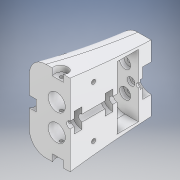
# Autodesk Inventor part: AA016
Saved by Autodesk Inventor 2017 SP1 (Build 210196100, 196)
## iProperties
Created: 2017-09-29
Part Number: AA016
Material: ABS Plastic
Document SubType Name: Modeling
Designer: Zach
Density: 1.06 g/cm^3
Appearance: CR White
Author: Zach
Autodesk Inventor part; units mm, degrees
sketch "Sketch1" plane through (0, 0, 0) normal (0, 0, 1) x (1, 0, 0)
  line L0 (0, 0) -> (70, 0)
  line L1 (70, 0) -> (70, 77.5)
  line L2 (70, 77.5) -> (0, 77.5)
  line L3 (0, 77.5) -> (0, 0)
  dimension "d0" = 70
  dimension "d1" = 77.5
  constraints: 8 end point, 2 parallel, 1 horizontal, 1 perpendicular
  measures "d0" distance of L2.end L1.end
  measures "d1" distance of L1.end L0.end
extrude "Extrusion1" add sketch "Sketch1" along normal blind 95
sketch "Sketch3" plane through (0, 0, 95) normal (0, 0, 1) x (1, 0, 0)
  line L0 (0, 0) -> (70, 0) projected
  line L1 (70, 77.5) -> (0, 77.5) projected
  line L2 (70, 0) -> (35, 0)
  line L3 (35, 0) -> (35, 77.5)
  line L4 (35, 77.5) -> (70, 77.5)
  line L5 (70, 77.5) -> (70, 0)
  constraints: 8 end point, 2 parallel, 1 horizontal, 1 midpoint, 1 perpendicular
extrude "Extrusion3" cut sketch "Sketch3" against normal through all
sketch "Sketch4" plane through (0, 77.5, 95) normal (0, 1, 0) x (1, 0, 0)
  line L0 (0, 95) -> (0, 0) projected
  line L1 (0, 0) -> (-12.5, 0)
  line L2 (35, 95) -> (0, 95) projected
  arc A0 (-12.5, 0) -> (0, 95) centre (-1145.4326, 197.3924) ccw
  line L3 (-12.5, -10) -> (35, -10) construction
  dimension "d9" = 1150
  dimension "d54" = 47.5
  dimension "d55" = 10
  constraints: 4 end point, 2 horizontal, 2 point on circle, 2 vertical alignment, 1 centre point
  measures "d9" radius of A0
  measures "d54" distance of L3.start L3.end
  measures "d55" distance between parallel lines of L1 L3
extrude "Extrusion4" add sketch "Sketch4" against normal blind 77.5
sketch "Sketch5" plane through (35, 0, 95) normal (1, 0, 0) x (0, 0, -1)
  line L0 (0, 77.5) -> (0, 86.25)
  line L1 (0, 0) -> (0, -8.75)
  line L2 (0, 0) -> (0, 77.5) projected
  line L3 (95, 77.5) -> (95, 0) projected
  arc A0 (0, 86.25) -> (95, 77.5) centre (152.8838, 1226.0423) ccw
  arc A1 (95, 0) -> (0, -8.75) centre (152.8838, -1148.5423) ccw
  line L4 (0, 77.5) -> (95, 77.5) projected
  line L5 (95, 0) -> (0, 0) projected
  line L6 (-10, 86.25) -> (-10, -8.75) construction
  point P0 (-10, 38.75)
  point P1 (0, 38.75)
  dimension "d14" = 1150
  dimension "d15" = 1150
  dimension "d52" = 10
  dimension "d53" = 95
  constraints: 6 end point, 4 point on circle, 3 horizontal alignment, 3 vertical, 2 centre point, 2 midpoint
  measures "d14" radius of A0
  measures "d15" radius of A1
  measures "d52" distance between parallel lines of L2 L6
  measures "d53" distance of L6.start L6.end
extrude "Extrusion5" add sketch "Sketch5" against normal blind 55 contours L0 A0 L4 | L5 A1 L1
sketch "Sketch6" plane through (-20, 0, 0) normal (0, 1, 0) x (1, 0, 0)
  line L0 (20, 0) -> (0, 0) projected
  line L1 (0, -95) -> (0, 0) projected
  arc A0 (7.5, -95) -> (20, 0) centre (-1125.4326, 102.3924) ccw projected
  line L2 (7.5, -95) -> (0, -95) projected
extrude "Extrusion6" cut sketch "Sketch6" along normal through all both and the other way through all
fillet "Fillet3" radius 19.35 2 edges at (-5.299, 80.9203, 47.9253) (-5.299, -3.4203, 47.9253)
sketch "Sketch27" plane through (0, 0, 0) normal (0, 0, -1) x (-1, 0, 0)
  line L0 (-35, 77.5) -> (-35, 0) projected
  circle A0 centre (-35, 38.75) radius 16.5
  point P0 (0, 0)
  dimension "d95" = 33
  constraints: 1 centre point, 1 midpoint
  measures "d95" diameter of A0
extrude "Extrusion24" cut sketch "Sketch27" against normal blind 10
sketch "Sketch28" plane through (0, 0, 10) normal (0, 0, -1) x (-1, 0, 0)
  line L0 (-35, 22.25) -> (-35, 55.25) projected
  circle A0 centre (-35, 38.75) radius 2.5
  point P0 (0, 0)
  dimension "d98" = 5
  constraints: 1 centre point, 1 midpoint
  measures "d98" diameter of A0
extrude "Extrusion25" cut sketch "Sketch28" against normal through all
sketch "Sketch29" plane through (0, 0, 10) normal (0, 0, -1) x (-1, 0, 0)
  arc A0 (-35, 36.25) -> (-35, 41.25) centre (-35, 38.75) ccw projected
  circle A1 centre (-35, 38.75) radius 5
  point P0 (0, 0)
  dimension "d101" = 10
  constraints: 1 centre point, 1 coincident
  measures "d101" diameter of A1
extrude "Extrusion26" cut sketch "Sketch29" against normal blind 3
sketch "Sketch30" plane through (0, 0, 10) normal (0, 0, -1) x (-1, 0, 0)
  circle A0 centre (-26.5, 38.75) radius 2
  arc A1 (-35, 36.25) -> (-35, 41.25) centre (-35, 38.75) ccw projected
  point P0 (0, 0)
  dimension "d104" = 4
  dimension "d105" = 8.5
  constraints: 1 centre point, 1 horizontal alignment
  measures "d104" diameter of A0
  measures "d105" distance of A0.centre A1.centre
extrude "Extrusion27" cut sketch "Sketch30" against normal through all
sketch "Sketch31" plane through (0, 0, 95) normal (0, 0, 1) x (1, 0, 0)
  arc A0 (35, 55.25) -> (35, 22.25) centre (35, 38.75) ccw projected
  circle A1 centre (35, 38.75) radius 16.5
  point P0 (0, 0)
  constraints: 1 coincident, 1 vertical alignment, 2 other
extrude "Extrusion28" cut sketch "Sketch31" against normal blind 80
sketch "Sketch32" plane through (0, 0, 15) normal (0, 0, 1) x (1, 0, 0)
  circle A0 centre (26.5, 38.75) radius 2 projected
  circle A1 centre (26.5, 38.75) radius 4.5
  point P0 (0, 0)
  dimension "d110" = 9
  constraints: 1 centre point, 1 coincident
  measures "d110" diameter of A1
extrude "Extrusion29" cut sketch "Sketch32" against normal blind 3
sketch "Sketch35" plane through (0, 0, 15) normal (0, 0, 1) x (1, 0, 0)
  arc A0 (35, 41.25) -> (35, 36.25) centre (35, 38.75) ccw projected
  arc A1 (35, 55.25) -> (35, 22.25) centre (35, 38.75) ccw projected
  line L0 (35, 22.25) -> (35, 0) projected
  line L1 (19.3399, 0) -> (35, 0) projected
  spline S0 degree 7 poles (0, 19.2875) (0, 18.3038) (0.0584, 17.2982) (0.18, 16.2758) (0.3689, 15.2432) (0.6283, 14.2079) (0.9599, 13.1783) (1.7682, 11.1451) (2.2454, 10.1417) (2.7951, 9.1614) (3.4157, 8.2132) (4.1036, 7.3058) (4.8535, 6.4473) (6.4663, 4.8388) (7.3295, 4.0892) (8.2417, 3.4018) (9.195, 2.7819) (10.1805, 2.2331) (11.1893, 1.7569) (13.2283, 0.9527) (14.2584, 0.6237) (15.2941, 0.3662) (16.3271, 0.1787) (17.3498, 0.058) (18.3558, 0) (19.3399, 0) knots 0 0 0 0 0 0 0 0 0.249652 0.249652 0.249652 0.249652 0.249652 0.249652 0.499923 0.499923 0.499923 0.499923 0.499923 0.499923 0.750832 0.750832 0.750832 0.750832 0.750832 0.750832 1 1 1 1 1 1 1 1
  line L2 (0, 58.2125) -> (0, 19.2875) projected
  spline S1 degree 7 poles (19.3399, 77.5) (18.3558, 77.5) (17.3498, 77.442) (16.3271, 77.3213) (15.2941, 77.1338) (14.2584, 76.8763) (13.2283, 76.5473) (11.1893, 75.7431) (10.1805, 75.2669) (9.195, 74.7181) (8.2417, 74.0982) (7.3295, 73.4108) (6.4663, 72.6612) (4.8535, 71.0527) (4.1036, 70.1942) (3.4157, 69.2868) (2.7951, 68.3386) (2.2454, 67.3583) (1.7682, 66.3549) (0.9599, 64.3217) (0.6283, 63.2921) (0.3689, 62.2568) (0.18, 61.2242) (0.0584, 60.2018) (0, 59.1962) (0, 58.2125) knots 0 0 0 0 0 0 0 0 0.249168 0.249168 0.249168 0.249168 0.249168 0.249168 0.500077 0.500077 0.500077 0.500077 0.500077 0.500077 0.750348 0.750348 0.750348 0.750348 0.750348 0.750348 1 1 1 1 1 1 1 1
  line L3 (35, 77.5) -> (19.3399, 77.5) projected
  line L4 (35, 77.5) -> (35, 55.25) projected
  line L5 (2, 58.2125) -> (2, 19.2875)
  line L6 (19.3399, 2) -> (33, 2)
  line L7 (33, 2) -> (33, 20.3584) construction
  arc A2 (33, 57.1416) -> (33, 20.3584) centre (35, 38.75) ccw construction
  line L8 (33, 57.1416) -> (33, 75.5) construction
  line L9 (33, 75.5) -> (19.3399, 75.5)
  line L10 (33, 75.5) -> (35, 75.5)
  line L11 (33, 2) -> (35, 2)
  spline S2 degree 5 poles (2, 19.2875) (2.0001, 16.57) (2.5325, 13.8525) (3.6013, 11.2745) (6.6986, 6.6755) (11.3083, 3.5933) (13.8938, 2.53) (16.6168, 2.0001) (19.3399, 2) knots 0 0 0 0 0 0 0.499487 0.499487 0.499487 1 1 1 1 1 1
  spline S3 degree 5 poles (19.3399, 75.5) (16.6168, 75.4999) (13.8938, 74.97) (11.3083, 73.9067) (6.6986, 70.8245) (3.6013, 66.2255) (2.5325, 63.6475) (2.0001, 60.93) (2, 58.2125) knots 0 0 0 0 0 0 0.500513 0.500513 0.500513 1 1 1 1 1 1
  point P0 (0, 0)
  dimension "d120" = 2
  constraints: 14 end point, 3 parallel, 2 perpendicular, 2 point on circle, 2 point on line, 1 centre point, 12 other
extrude "Extrusion30" cut sketch "Sketch35" along normal blind 25 contours A1 L0 L11 L6 S2 L5 S3 L9 L10 L4
sketch "Sketch39" plane through (0, 0, 95) normal (0, 0, 1) x (1, 0, 0)
  arc A0 (35, 55.25) -> (35, 22.25) centre (35, 38.75) ccw projected
  arc A1 (35, 55.25) -> (35, 22.25) centre (35, 38.75) ccw projected
  line L0 (35, 22.25) -> (35, 22.25)
  line L1 (35, 43.75) -> (35, 55.25) projected
  line L2 (35, 55.25) -> (35, 22.25)
  point P0 (0, 0)
  constraints: 4 end point, 1 collinear
extrude "Extrusion33" add sketch "Sketch39" against normal blind 55
ref_plane "Work Plane4" through (0, 0, 45) normal (0, 0, -1) x (-1, 0, 0)
sketch "Sketch42" plane through (0, 0, 45) normal (0, 0, -1) x (-1, 0, 0)
  line L0 (-35, 2) -> (-35, 75.5) projected
  circle A0 centre (-35, 38.75) radius 11.5
  point P0 (0, 0)
  dimension "d136" = 23
  constraints: 1 centre point, 1 midpoint
  measures "d136" diameter of A0
extrude "Extrusion35" cut sketch "Sketch42" against normal blind 9
sketch "Sketch43" plane through (0, 0, 40) normal (0, 0, -1) x (-1, 0, 0)
  circle A0 centre (-35, 38.75) radius 4
  line L0 (-35, 86.25) -> (-35, -8.75) projected
  point P0 (0, 0)
  point P1 (-35, 38.75)
  dimension "d139" = 8
  constraints: 1 centre point, 1 coincident, 1 midpoint
  measures "d139" diameter of A0
extrude "Extrusion36" cut sketch "Sketch43" against normal through all
ref_plane "Work Plane5" through (0, 0, 90) normal (0, 0, 1) x (1, 0, 0)
sketch "Sketch45" plane through (0, 0, 90) normal (0, 0, 1) x (1, 0, 0)
  circle A0 centre (35, 38.75) radius 11.5
  arc A1 (35, 41.25) -> (35, 36.25) centre (35, 38.75) ccw projected
  point P0 (0, 0)
  dimension "d143" = 23
  constraints: 1 centre point, 1 coincident
  measures "d143" diameter of A0
extrude "Extrusion37" cut sketch "Sketch45" against normal blind 9
sketch "Sketch46" plane through (35, 55.25, 0) normal (1, 0, 0) x (0, 0, -1)
  line L0 (-67.5, 13.5) -> (-67.5, -46.5) construction
  line L1 (0, 0) -> (0, -33) projected
  circle A0 centre (-67.5, 13.5) radius 2.5
  circle A1 centre (-67.5, -46.5) radius 2.5
  line L2 (-81, -12.5) -> (-54, -12.5) projected
  point P0 (0, -55.25)
  point P1 (-67.5, -16.5)
  point P2 (0, -16.5)
  point P3 (-67.5, -12.5)
  dimension "d146" = 60
  dimension "d147" = 5
  dimension "d148" = 5
  constraints: 3 midpoint, 2 centre point, 2 coincident, 2 end point, 1 horizontal alignment, 1 vertical, 1 vertical alignment
  measures "d146" distance of L0.start L0.end
  measures "d147" diameter of A0
  measures "d148" diameter of A1
extrude "Extrusion38" cut sketch "Sketch46" against normal through all
sketch "Sketch48" plane through (0, 0, 95) normal (0, 0, 1) x (1, 0, 0)
  line L0 (50.5, 54.25) -> (19.5, 54.25) construction
  line L1 (19.5, 54.25) -> (19.5, 23.25) construction
  line L2 (19.5, 23.25) -> (50.5, 23.25) construction
  line L3 (50.5, 23.25) -> (50.5, 54.25) construction
  arc A0 (35, 42.75) -> (35, 34.75) centre (35, 38.75) ccw projected
  circle A1 centre (19.5, 54.25) radius 2.5
  circle A2 centre (19.5, 23.25) radius 2.5
  point P0 (0, 0)
  point P1 (50.5, 38.75)
  point P2 (35, 54.25)
  dimension "d157" = 31
  dimension "d158" = 31
  dimension "d159" = 5
  dimension "d160" = 5
  constraints: 8 end point, 2 centre point, 2 coincident, 2 midpoint, 2 parallel, 1 horizontal, 1 horizontal alignment, 1 perpendicular, 1 vertical alignment
  measures "d157" distance of L2.end L1.end
  measures "d158" distance of L1.end L0.end
  measures "d159" diameter of A1
  measures "d160" diameter of A2
extrude "Extrusion40" cut sketch "Sketch48" against normal through all
sketch "Sketch51" plane through (0, 0, 15) normal (0, 0, 1) x (1, 0, 0)
  circle A0 centre (19.5, 54.25) radius 2.5 projected
  circle A1 centre (19.5, 23.25) radius 2.5 projected
  circle A2 centre (19.5, 54.25) radius 6.5
  circle A3 centre (19.5, 23.25) radius 6.5
  point P0 (0, 0)
  dimension "d164" = 13
  dimension "d165" = 13
  constraints: 2 centre point, 2 coincident
  measures "d164" diameter of A2
  measures "d165" diameter of A3
extrude "Extrusion41" cut sketch "Sketch51" against normal blind 5
ref_plane "Work Plane6" through (-12.5, 10.3275, 95) normal (1, 0, 0) x (0, 1, 0)
sketch "Sketch52" plane through (-12.5, 10.3275, 95) normal (1, 0, 0) x (0, 1, 0)
  circle A0 centre (-1.5775, -27.5) radius 2.5 projected
  circle A1 centre (58.4225, -27.5) radius 2.5 projected
  circle A2 centre (58.4225, -27.5) radius 2.5 projected
  circle A3 centre (-1.5775, -27.5) radius 10
  circle A4 centre (58.4225, -27.5) radius 10
  point P0 (-10.3275, -95)
  dimension "d168" = 20
  dimension "d169" = 20
  constraints: 2 centre point, 2 coincident, 2 other
  measures "d168" diameter of A3
  measures "d169" diameter of A4
extrude "Extrusion42" cut sketch "Sketch52" along normal blind 42.5
sketch "Sketch53" plane through (0, 0, 95) normal (0, 0, 1) x (1, 0, 0)
  circle A0 centre (19.5, 54.25) radius 2.5 projected
  circle A1 centre (19.5, 23.25) radius 2.5 projected
  circle A2 centre (19.5, 54.25) radius 2.5 projected
  circle A3 centre (19.5, 54.25) radius 10
  circle A4 centre (19.5, 23.25) radius 2.5 projected
  circle A5 centre (19.5, 23.25) radius 10
  point P0 (0, 0)
  dimension "d172" = 20
  dimension "d173" = 20
  constraints: 2 centre point, 2 coincident
  measures "d172" diameter of A3
  measures "d173" diameter of A5
extrude "Extrusion43" cut sketch "Sketch53" against normal blind 80
ref_plane "Work Plane7" through (35, 86.25, 95) normal (0, 1, 0) x (-1, 0, 0)
ref_plane "Work Plane8" through (35, -8.75, 95) normal (0, 1, 0) x (-1, 0, 0)
ref_plane "Work Plane9" through (-12.5, 10.3275, 95) normal (1, 0, 0) x (0, 1, 0)
sketch "Sketch54" plane through (35, 86.25, 95) normal (0, 1, 0) x (-1, 0, 0)
  line L0 (0, 0) -> (28.3069, 0) projected
  circle A0 centre (14.1535, -4) radius 7.5
  point P0 (35, -95)
  point P1 (14.1535, 0)
  dimension "d176" = 15
  dimension "d177" = 4
  constraints: 1 centre point, 1 midpoint, 1 vertical alignment
  measures "d176" diameter of A0
  measures "d177" distance from line of L0 A0.centre
extrude "Extrusion44" cut sketch "Sketch54" against normal blind 8
sketch "Sketch55" plane through (35, -8.75, 95) normal (0, 1, 0) x (-1, 0, 0)
  circle A0 centre (14.1535, -4) radius 7.5
  line L0 (0, 0) -> (28.3069, 0) projected
  point P0 (35, -95)
  point P1 (14.1535, 0)
  dimension "d180" = 15
  dimension "d181" = 4
  constraints: 1 centre point, 1 midpoint, 1 vertical alignment
  measures "d180" diameter of A0
  measures "d181" distance from line of L0 A0.centre
extrude "Extrusion45" cut sketch "Sketch55" along normal blind 8
sketch "Sketch56" plane through (-12.5, 10.3275, 95) normal (1, 0, 0) x (0, 1, 0)
  line L0 (56.8449, 0) -> (0, 0) projected
  circle A0 centre (28.4225, -4) radius 7.5
  point P0 (-10.3275, -95)
  point P1 (28.4225, 0)
  dimension "d184" = 15
  dimension "d185" = 4
  constraints: 1 centre point, 1 midpoint, 1 vertical alignment
  measures "d184" diameter of A0
  measures "d185" distance from line of L0 A0.centre
extrude "Extrusion46" cut sketch "Sketch56" along normal blind 8
sketch "Sketch57" plane through (35, 78.25, 95) normal (0, 1, 0) x (1, 0, 0)
  circle A0 centre (-14.1535, 4) radius 2
  arc A1 (-7.8092, 0) -> (-20.4978, 0) centre (-14.1535, 4) ccw projected
  point P0 (-35, 95)
  dimension "d188" = 4
  constraints: 1 centre point, 1 concentric, 1 horizontal alignment
  measures "d188" diameter of A0
extrude "Extrusion47" cut sketch "Sketch57" against normal through all
sketch "Sketch58" plane through (-4.5, 10.3275, 95) normal (-1, 0, 0) x (0, 0, 1)
  circle A0 centre (-4, 28.4225) radius 2
  arc A1 (0, 34.7667) -> (0, 22.0782) centre (-4, 28.4225) ccw projected
  point P0 (-95, -10.3275)
  dimension "d191" = 4
  constraints: 1 centre point, 1 concentric, 1 vertical alignment
  measures "d191" diameter of A0
extrude "Extrusion48" cut sketch "Sketch58" against normal through all
body "Solid1"
